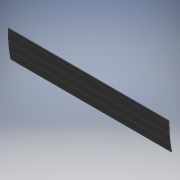
# Autodesk Inventor part: base
Saved by Autodesk Inventor 2018.1 (Build 221171000, 171)
## iProperties
Created: 2017-10-18
Part Number: base
Material: CFRP
Document SubType Name: Modeling
Designer: kuwano
Density: 1.43 g/cm^3
Appearance: カーボンファイバー
Mass: 2365.86 g
Surface Area: 6778.95 cm^2
Volume: 1654.45 cm^3
Author: kuwano
Autodesk Inventor part; units mm, degrees
ref_plane "YZ Plane" through (0, 0, 0) normal (1, 0, 0) x (0, 1, 0)
ref_plane "XZ Plane" through (0, 0, 0) normal (0, 1, 0) x (-1, 0, 0)
ref_plane "XY Plane" through (0, 0, 0) normal (0, 0, 1) x (1, 0, 0)
sketch "スケッチ2" plane through (0, 0, 0) normal (1, 0, 0) x (0, 1, 0)
  arc A0 (-5, 100) -> (15.099, -100.9901) centre (1010, 100) ccw
  arc A1 (0, 100) -> (20, -100) centre (1010, 100) ccw
  line L0 (0, 100) -> (-5, 100)
  line L1 (20, -100) -> (15.099, -100.9901)
  line L2 (0, -141.7896) -> (0, 140.2983) projected
  line L3 (-214.0147, 0) -> (1214.0025, 0) projected
  point P0 (0, 0)
  dimension "d5" = 5
  dimension "d6" = 100
  dimension "d9" = 20
  dimension "d10" = 100
  constraints: 4 end point, 4 line through centre, 4 point on circle, 2 centre point, 1 concentric, 1 point on line, 1 tangent
  measures "d5" radial gap between concentric circles of A0 A1
  measures "d6" distance from line of L3 L0.start
  measures "d9" distance from line of L2 L1.start
  measures "d10" distance from line of L3 L1.start
extrude "押し出し2" add sketch "スケッチ2" along normal mid plane 1370
sketch "スケッチ3" plane through (-685, -5, 100) normal (0, 0, 1) x (1, 0, 0)
  line L0 (0, 0) -> (1370, 0) projected
  line L1 (1370, 5) -> (1370, 0) projected
  line L2 (0, 0) -> (1370, 0)
  line L3 (1370, 0) -> (1370, 5)
  line L4 (1370, 5) -> (0, 5)
  line L5 (0, 5) -> (0, 0)
  point P0 (685, 5)
  constraints: 8 end point, 2 parallel, 1 horizontal, 1 perpendicular
extrude "押し出し3" add sketch "スケッチ3" along normal blind 30
sketch "スケッチ4" plane through (685, 20, -100) normal (0, 0.198, -0.9802) x (-1, 0, 0)
  line L0 (0, 15.099) -> (0, -5) projected
  line L1 (1370, 0) -> (0, 0) projected
  line L2 (0, -5) -> (1370, -5)
  line L3 (1370, -5) -> (1370, 0)
  line L4 (1370, 0) -> (0, 0)
  line L5 (0, 0) -> (0, -5)
  point P0 (685, 0.198)
  constraints: 8 end point, 2 parallel, 1 horizontal, 1 perpendicular
extrude "押し出し4" add sketch "スケッチ4" along normal blind 10
sketch "スケッチ5" plane through (685, 0, 0) normal (1, 0, 0) x (0, 0, -1)
  line L0 (-40.0262, -3.2266) -> (-30.0467, -2.5866)
  line L1 (31.9441, 3.6125) -> (41.8527, 4.9613)
  arc A0 (-100, -5) -> (100.9901, 15.099) centre (-100, 1010) ccw projected
  point P0 (0, 0)
  dimension "d15" = 10
  dimension "d16" = 10
  dimension "d17" = 60
  dimension "d18" = 60
  constraints: 4 end point, 4 point on circle
  measures "d15" distance of L1.start L1.end
  measures "d16" distance of L0.start L0.end
  measures "d17" distance of A0.end L1.end
  measures "d18" distance of A0.start L0.start
extrude "押し出し5" cut sketch "スケッチ5" against normal through all
